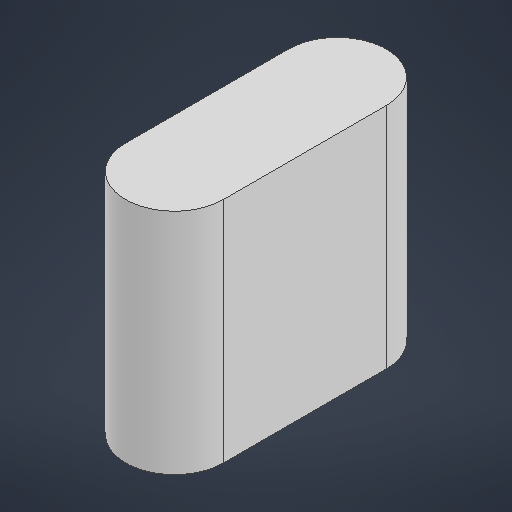
# Autodesk Inventor part: paletas
Saved by Autodesk Inventor 2025.3 (Build 293356000, 356)
## iProperties
Created: 2025-10-02
Part Number: paletas
Material: Generic
Document SubType Name: Modeling
Designer: sophi
Density: 1 g/cm^3
Appearance: Default
Author: sophi
Autodesk Inventor part; units mm, degrees
ref_plane "YZ Plane" through (0, 0, 0) normal (1, 0, 0) x (0, 1, 0)
ref_plane "XZ Plane" through (0, 0, 0) normal (0, 1, 0) x (-1, 0, 0)
ref_plane "XY Plane" through (0, 0, 0) normal (0, 0, 1) x (1, 0, 0)
sketch "Sketch1" plane through (0, 0, 0) normal (0, 1, 0) x (-1, 0, 0)
  line L0 (0, 5) -> (0, -5) construction
  line L1 (3, 5) -> (3, -5)
  line L2 (-3, -5) -> (-3, 5)
  arc A0 (3, 5) -> (-3, 5) centre (0, 5) ccw
  arc A1 (-3, -5) -> (3, -5) centre (0, -5) ccw
  line L3 (0, 30.2784) -> (0, -34.8413) construction
  line L4 (24.1166, 0) -> (-17.2731, 0) construction
  point P0 (0, 0)
  dimension "d0" = 10
  dimension "d1" = 3
  constraints: 12 end point, 4 point on circle, 4 tangent, 2 centre point, 2 point on line, 2 vertical, 1 horizontal, 1 midpoint, 1 parallel
  measures "d0" distance of L0.start L0.end
  measures "d1" radius of A1
extrude "Extrusion1" add sketch "Sketch1" along normal blind 14
ref_plane "Work Plane2" through (0, 14, -8) normal (0, 0, -1) x (-1, 0, 0)
sketch "Sketch3" plane through (0, 14, -8) normal (0, 0, -1) x (-1, 0, 0)
  circle A0 centre (0, -7) radius 1.5
  line L0 (3, -14) -> (3, 0) projected
  line L1 (3, 0) -> (-3, 0) projected
  line L2 (-3, -14) -> (3, -14) projected
  line L3 (3, -14) -> (3, 0) projected
  line L4 (-3, 0) -> (3, 0) projected
  line L5 (-3, -14) -> (-3, 0) projected
  point P0 (0, -14)
  dimension "d12" = 3
  dimension "d13" = 7
  dimension "d14" = 3
  constraints: 1 centre point
  measures "d12" diameter of A0
  measures "d13" distance from line of L1 A0.centre
  measures "d14" distance from line of A0.centre L0
extrude "Extrusion3" cut sketch "Sketch3" against normal blind 5 contours A0
body "Solid1"
